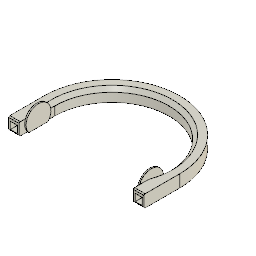
Headset without loops (Autodesk Fusion 360 design; units mm, degrees)
Autodesk Fusion 360 part; units mm, degrees
note: some values were not read from the file. Set by a fixed rule: which face or edge a step refers to.
sketch "Sketch1" plane through (0, 0, 0) normal (0, 0, 1) x (1, 0, 0)
  arc A0 (177.6758, 0) -> (2.3242, 0) centre (90, 0) ccw
  line L0 (2.3242, 0) -> (2.3242, -50)
  line L1 (177.6758, 0) -> (177.6758, -50)
  dimension "d1" = 87.6758
  dimension "d2" = 50
  dimension "d3" = 50
  constraint vertical L0
  constraint vertical L1
  measures "d1" radius of A0
  measures "d2" distance of A0.end L0.end
  measures "d3" distance of A0.start L1.end
ref_plane "WorkPlane1" through (0, 0, 15) normal (0, 0, 1) x (1, 0, 0)
sketch "Sketch2" plane through (0, 0, 15) normal (0, 0, 1) x (1, 0, 0)
  line L0 (2.3242, 0) -> (2.3242, -50)
  arc A0 (177.6758, 0) -> (2.3242, 0) centre (90, 0) ccw
  line L1 (177.6758, 0) -> (177.6758, -50)
  line L2 (2.3242, 0) -> (177.6758, 0) construction
  dimension "d5" = 87.6758
  dimension "d6" = 50
  dimension "d7" = 50
  constraint vertical L0
  constraint vertical L1
  constraint perpendicular L1 L2
  measures "d5" radius of A0
  measures "d6" distance of L0.end L0.start
  measures "d7" distance of A0.start L1.end
ref_plane "WorkPlane2" through (90, 0, 15) normal (0, -1, 0) x (1, 0, 0)
ref_plane "WorkPlane3" through (90, -50, 15) normal (0, -1, 0) x (1, 0, 0)
sketch "Sketch3" plane through (90, -50, 15) normal (0, -1, 0) x (1, 0, 0)
  line L0 (-80.1758, 10) -> (-95.1758, 10)
  line L1 (-95.1758, 10) -> (-95.1758, -7.5)
  line L2 (-95.1758, -7.5) -> (-80.1758, -7.5)
  line L3 (-80.1758, -7.5) -> (-80.1758, 10)
  line L4 (-82.6758, 5) -> (-92.6758, 5)
  line L5 (-92.6758, 5) -> (-92.6758, -5)
  line L6 (-92.6758, -5) -> (-82.6758, -5)
  line L7 (-82.6758, -5) -> (-82.6758, 5)
  line L8 (-82.6758, 5) -> (-92.6758, -5) construction
  line L9 (-92.6758, 5) -> (-82.6758, -5) construction
  point P0 (-87.6758, 0)
  point P1 (87.6758, 0)
  point P2 (-87.6758, 0)
  point P3 (-87.6758, 0)
  dimension "d10" = 15
  dimension "d18" = 10
  dimension "d19" = 10
  dimension "d26" = 5
  constraint perpendicular L0 L1
  constraint parallel L1 L3
  constraint coincident P3 P2
  constraint horizontal L4
  constraint perpendicular L4 L5
  constraint parallel L4 L6
  constraint parallel L5 L7
  constraint coincident L8 P3
  constraint coincident L9 P3
  measures "d10" distance of L1.end L2.end
  measures "d18" distance of L5.end L6.end
  measures "d19" distance of L4.end L5.end
  measures "d26" distance of L0 L4
sweep "Sweep2" add profiles "Sketch3" path "Sketch2" along L1 A0 L0 section 1
chamfer "Chamfer1" distance 5 angle 45 3 edges at (9.8242, -25, 25) (90, 80.1758, 25) (170.1758, -25, 25)
delete_face "DeleteFace1" 1 faces at (6.4909, -33.3333, 23.3333)
delete_face "DeleteFace2" 1 faces at (173.5091, -16.6667, 23.3333)
sketch "Sketch4" plane through (9.8242, 0, 0) normal (1, 0, 0) x (0, 1, 0)
  line L0 (-28.7534, 25) -> (-50, 25)
  line L1 (-50, 25) -> (-50, 7.5)
  line L2 (-50, 7.5) -> (0, 7.5)
  line L3 (0, 7.5) -> (0, 20)
  spline S0 degree 2 poles (0, 20) (-13.942, 20) (-28.7534, 25) knots 3.215758 3.215758 3.215758 6.160193 6.160193 6.160193 weights 1.037418 1.037418 1.006048
  circle A0 centre (-25, 18.75) radius 17.5
  line L4 (-50, 16.25) -> (0, 16.25)
  dimension "d28" = 35
  constraint coincident L1 L4.start
  constraint coincident L3 L4.end
  constraint perpendicular L3 L4
  constraint midpoint L1 L4.start
  measures "d28" diameter of A0
extrude "Extrude1" add sketch "Sketch4" along normal blind 2 contours L0 S0 A0 L4 | L0 S0 A0 | L2 A0 L4 | L2 A0
sketch "Sketch5" plane through (170.1758, 0, 0) normal (-1, 0, 0) x (0, -1, 0)
  spline S0 degree 2 poles (0, 20) (13.942, 20) (28.7534, 25) knots 2.91849 2.91849 2.91849 5.836979 5.836979 5.836979 weights 1.031181 1.031181 1
  line L0 (0, 20) -> (0, 7.5)
  line L1 (0, 7.5) -> (50, 7.5)
  line L2 (50, 7.5) -> (50, 25)
  line L3 (50, 25) -> (28.7534, 25)
  circle A0 centre (25, 18.75) radius 17.5
  line L4 (50, 25) -> (50, 7.5)
  line L5 (28.7534, 25) -> (50, 25)
  spline S1 degree 2 poles (0, 20) (13.942, 20) (28.7534, 25) knots 2.91849 2.91849 2.91849 5.836979 5.836979 5.836979 weights 1.031181 1.031181 1
  line L6 (0, 20) -> (0, 7.5)
  line L7 (0, 7.5) -> (50, 7.5)
  line L8 (0, 13.75) -> (50, 13.75)
  point P0 (50, 0)
  dimension "d31" = 35
  constraint horizontal L8
  constraint midpoint L6 L8.start
  constraint coincident L4 L8.end
  measures "d31" diameter of A0
extrude "Extrude2" add sketch "Sketch5" along normal blind 2 contours S0 L3 A0 L5 S1 | S0 L3 A0 L5 S1 L8 | L1 A0 L7 L8 | L1 A0 L7
delete_face "DeleteFace3" 1 faces at (170.1758, -21.1224, 6.8921)
delete_face "DeleteFace4" 1 faces at (9.8242, -28.8776, 6.8921)
sketch "Sketch6" plane through (0, 0, 25) normal (0, 0, 1) x (-1, 0, 0)
  arc A0 (-170.1758, 28.7534) -> (-9.8242, 28.7534) centre (-90, 0) ccw
  line L0 (-170.1758, 28.7534) -> (-170.1758, 41.3459)
  line L1 (-170.1758, 41.3459) -> (-170.1758, 50)
  line L2 (-185.1758, 50) -> (-185.1758, 0)
  arc A1 (-185.1758, 0) -> (5.1758, 0) centre (-90, 0) ccw
  line L3 (5.1758, 0) -> (5.1758, 50)
  line L4 (-9.8242, 50) -> (-9.8242, 41.3459)
  line L5 (-9.8242, 41.3459) -> (-9.8242, 28.7534)
  line L6 (10, -95.1758) -> (-190, -95.1758) construction
  constraint horizontal L6
  constraint midpoint A1 L6
ref_plane "WorkPlane4" through (90, 95.1758, 25) normal (0, -1, 0) x (1, 0, 0)
fillet "Fillet5" radius 1.5 4 edges at (2.3242, -50, 25) (2.3242, -50, 7.5) (177.6758, -50, 7.5) (177.6758, -50, 25)
sketch "Sketch7" plane through (90, 95.1758, 25) normal (0, -1, 0) x (1, 0, 0)
  line L0 (-95.1758, -17.5) -> (95.1758, -17.5)
  line L1 (95.1758, 0) -> (-95.1758, 0)
  line L2 (-95.1758, -17.5) -> (-95.1758, 0)
  line L3 (95.1758, -17.5) -> (95.1758, 0)
  circle A0 centre (0, -10) radius 5
  line L4 (95.1758, -5) -> (-95.1758, -5) construction
  line L5 (-100, 0) -> (100, 0)
  line L6 (0, 0) -> (0, -17.5) construction
  dimension "d40" = 10
  dimension "d43" = 5
  constraint coincident L3 L4.start
  constraint coincident L2 L4.end
  constraint perpendicular L2 L4
  constraint coincident L6.start origin
  constraint tangent A0 L4
  constraint coincident A0.centre L6
  measures "d40" diameter of A0
  measures "d43" distance of L4 L5
extrude "Extrude3" cut sketch "Sketch7" along normal blind 5 contours A0
